Autodesk Inventor part; units mm, degrees
(part 2 of 2)
  spline S197 degree 3 poles (37.725433, 80.080162) (38.103851, 80.500583) (38.500866, 80.903886) (39.329714, 81.67384) (39.761133, 82.040107) (40.208257, 82.386568) knots 0 0 0 0 0.5 0.5 1 1 1 1
  spline S198 degree 3 poles (40.208257, 82.386568) (40.397457, 82.29423) (40.586338, 82.201241) (40.963456, 82.013963) (41.151692, 81.919675) (41.339601, 81.824739) knots 0 0 0 0 0.5 0.5 1 1 1 1
  spline S199 degree 3 poles (41.339601, 81.824739) (41.333785, 81.259123) (41.302697, 80.69405) (41.190168, 79.56837) (41.108781, 79.008326) (41.002517, 78.452752) knots 0 0 0 0 0.5 0.5 1 1 1 1
  spline S200 degree 3 poles (42.079584, 77.880352) (42.480588, 78.279289) (42.899217, 78.660108) (43.769222, 79.383234) (44.220162, 79.725179) (44.685693, 80.046483) knots 0 0 0 0 0.5 0.5 1 1 1 1
  spline S201 degree 3 poles (44.685693, 80.046483) (44.869518, 79.943863) (45.05299, 79.84061) (45.419219, 79.632841) (45.601975, 79.528327) (45.78437, 79.423183) knots 0 0 0 0 0.5 0.5 1 1 1 1
  spline S202 degree 3 poles (45.78437, 79.423183) (45.747403, 78.858747) (45.685235, 78.296245) (45.510864, 77.178473) (45.39875, 76.623762) (45.262042, 76.074886) knots 0 0 0 0 0.5 0.5 1 1 1 1
  spline S203 degree 3 poles (46.305941, 75.444022) (46.728313, 75.820263) (47.167285, 76.177443) (48.075803, 76.851543) (48.544896, 77.168128) (49.02742, 77.463299) knots 0 0 0 0 0.5 0.5 1 1 1 1
  spline S204 degree 3 poles (49.02742, 77.463299) (49.205313, 77.350708) (49.382818, 77.237505) (49.737046, 77.009877) (49.913767, 76.895453) (50.090092, 76.780422) knots 0 0 0 0 0.5 0.5 1 1 1 1
  spline S205 degree 3 poles (50.090092, 76.780422) (50.022088, 76.21888) (49.929027, 75.660656) (49.693346, 74.554187) (49.550844, 74.006495) (49.384107, 73.465983) knots 0 0 0 0 0.5 0.5 1 1 1 1
  spline S206 degree 3 poles (50.391669, 72.778571) (50.834125, 73.130973) (51.292107, 73.463428) (52.23638, 74.086457) (52.722201, 74.37672) (53.220252, 74.644861) knots 0 0 0 0 0.5 0.5 1 1 1 1
  spline S207 degree 3 poles (53.220252, 74.644861) (53.391673, 74.522642) (53.562673, 74.399832) (53.903822, 74.153036) (54.073972, 74.029051) (54.243693, 73.904481) knots 0 0 0 0 0.5 0.5 1 1 1 1
  spline S208 degree 3 poles (54.243693, 73.904481) (54.144858, 73.347538) (54.021187, 72.795288) (53.724911, 71.703483) (53.552454, 71.164472) (53.356195, 70.633966) knots 0 0 0 0 0.5 0.5 1 1 1 1
  spline S209 degree 3 poles (54.324358, 69.892093) (54.785556, 70.219586) (55.261156, 70.526308) (56.238317, 71.096373) (56.73939, 71.359432) (57.251456, 71.59973) knots 0 0 0 0 0.5 0.5 1 1 1 1
  spline S210 degree 3 poles (57.251456, 71.59973) (57.415884, 71.468253) (57.579859, 71.336209) (57.906895, 71.070995) (58.069956, 70.937825) (58.232557, 70.804095) knots 0 0 0 0 0.5 0.5 1 1 1 1
  spline S211 degree 3 poles (58.232557, 70.804095) (58.103191, 70.253442) (57.949286, 69.708844) (57.593315, 68.635017) (57.391427, 68.106325) (57.166241, 67.587436) knots 0 0 0 0 0.5 0.5 1 1 1 1
  spline S212 degree 3 poles (58.092066, 66.793356) (58.570604, 67.094946) (59.062379, 67.375002) (60.06946, 67.890371) (60.584264, 68.125428) (61.108789, 68.337152) knots 0 0 0 0 0.5 0.5 1 1 1 1
  spline S213 degree 3 poles (61.108789, 68.337152) (61.265725, 68.196817) (61.422177, 68.055941) (61.734106, 67.773114) (61.889584, 67.631164) (62.044571, 67.488679) knots 0 0 0 0 0.5 0.5 1 1 1 1
  spline S214 degree 3 poles (62.044571, 67.488679) (61.885067, 66.945988) (61.701395, 66.410695) (61.28681, 65.358109) (61.056104, 64.841342) (60.802675, 64.335645) knots 0 0 0 0 0.5 0.5 1 1 1 1
  spline S215 degree 3 poles (61.683351, 63.49177) (62.177776, 63.76654) (62.684232, 64.01908) (63.718174, 64.478189) (64.245145, 64.684529) (64.780537, 64.867037) knots 0 0 0 0 0.5 0.5 1 1 1 1
  spline S216 degree 3 poles (64.780537, 64.867037) (64.929504, 64.718269) (65.077957, 64.568989) (65.373833, 64.269408) (65.521255, 64.119108) (65.668157, 63.968302) knots 0 0 0 0 0.5 0.5 1 1 1 1
  spline S217 degree 3 poles (65.668157, 63.968302) (65.479001, 63.435222) (65.266119, 62.91086) (64.794178, 61.882711) (64.535355, 61.379437) (64.254454, 60.88847) knots 0 0 0 0 0.5 0.5 1 1 1 1
  spline S218 degree 3 poles (65.087305, 59.997361) (65.596116, 60.244477) (66.115715, 60.468734) (67.173378, 60.870188) (67.710915, 61.047185) (68.255549, 61.199923) knots 0 0 0 0 0.5 0.5 1 1 1 1
  spline S219 degree 3 poles (68.255549, 61.199923) (68.396094, 61.043175) (68.536098, 60.885943) (68.815022, 60.570518) (68.95394, 60.412325) (69.092312, 60.253656) knots 0 0 0 0 0.5 0.5 1 1 1 1
  spline S220 degree 3 poles (69.092312, 60.253656) (68.874076, 59.731805) (68.632632, 59.219967) (68.104769, 58.219377) (67.818615, 57.731125) (67.511094, 57.256377) knots 0 0 0 0 0.5 0.5 1 1 1 1
  spline S221 degree 3 poles (68.293591, 56.320742) (68.815243, 56.539453) (69.346406, 56.734746) (70.424579, 57.077327) (70.97105, 57.224444) (71.523271, 57.346946) knots 0 0 0 0 0.5 0.5 1 1 1 1
  spline S222 degree 3 poles (71.523271, 57.346946) (71.654967, 57.182694) (71.786098, 57.017989) (72.047222, 56.687677) (72.177214, 56.522072) (72.306635, 56.356021) knots 0 0 0 0 0.5 0.5 1 1 1 1
  spline S223 degree 3 poles (72.306635, 56.356021) (72.059983, 55.846985) (71.790709, 55.349224) (71.208529, 54.379233) (70.895912, 53.907486) (70.562705, 53.4504) knots 0 0 0 0 0.5 0.5 1 1 1 1
  spline S224 degree 3 poles (71.292472, 52.473079) (71.82538, 52.662721) (72.366495, 52.828457) (73.461903, 53.111124) (74.015648, 53.227913) (74.573779, 53.319809) knots 0 0 0 0 0.5 0.5 1 1 1 1
  spline S225 degree 3 poles (74.573779, 53.319809) (74.696227, 53.148551) (74.818085, 52.976872) (75.060616, 52.632678) (75.181289, 52.460163) (75.301366, 52.287234) knots 0 0 0 0 0.5 0.5 1 1 1 1
  spline S226 degree 3 poles (75.301366, 52.287234) (75.027047, 51.792559) (74.730761, 51.310388) (74.09603, 50.37394) (73.757901, 49.920131) (73.40002, 49.482095) knots 0 0 0 0 0.5 0.5 1 1 1 1
  spline S227 degree 3 poles (74.07484, 48.466057) (74.617385, 48.626055) (75.166809, 48.76173) (76.276125, 48.983624) (76.835463, 49.069731) (77.397809, 49.130742) knots 0 0 0 0 0.5 0.5 1 1 1 1
  spline S228 degree 3 poles (77.397809, 49.130742) (77.510637, 48.952998) (77.622852, 48.774867) (77.846054, 48.417835) (77.95704, 48.238934) (78.067408, 48.059654) knots 0 0 0 0 0.5 0.5 1 1 1 1
  spline S229 degree 3 poles (78.067408, 48.059654) (77.766255, 47.580841) (77.443858, 47.115724) (76.758504, 46.215664) (76.395889, 45.781171) (76.014421, 45.363514) knots 0 0 0 0 0.5 0.5 1 1 1 1
  spline S230 degree 3 poles (76.632245, 44.311845) (77.182781, 44.441712) (77.738844, 44.546915) (78.858699, 44.707362) (79.421931, 44.762526) (79.986784, 44.792465) knots 0 0 0 0 0.5 0.5 1 1 1 1
  spline S231 degree 3 poles (79.986784, 44.792465) (80.089649, 44.608777) (80.191881, 44.424734) (80.395076, 44.055948) (80.496038, 43.871206) (80.596363, 43.686117) knots 0 0 0 0 0.5 0.5 1 1 1 1
  spline S232 degree 3 poles (80.596363, 43.686117) (80.269291, 43.224621) (79.921761, 42.777971) (79.187865, 41.917032) (78.801865, 41.503174) (78.397969, 41.107166) knots 0 0 0 0 0.5 0.5 1 1 1 1
  spline S233 degree 3 poles (78.956921, 40.023059) (79.513774, 40.122402) (80.074789, 40.196812) (81.201782, 40.295325) (81.767198, 40.319378) (82.332842, 40.318156) knots 0 0 0 0 0.5 0.5 1 1 1 1
  spline S234 degree 3 poles (82.332842, 40.318156) (82.425432, 40.12908) (82.517371, 39.939685) (82.699941, 39.560265) (82.790573, 39.370242) (82.880549, 39.179907) knots 0 0 0 0 0.5 0.5 1 1 1 1
  spline S235 degree 3 poles (82.880549, 39.179907) (82.528551, 38.73713) (82.156943, 38.310302) (81.376735, 37.4911) (80.968523, 37.099134) (80.543424, 36.725977) knots 0 0 0 0 0.5 0.5 1 1 1 1
  spline S236 degree 3 poles (81.041807, 35.612725) (81.603287, 35.681241) (82.167549, 35.724633) (83.298257, 35.760913) (83.86414, 35.753782) (84.428858, 35.721402) knots 0 0 0 0 0.5 0.5 1 1 1 1
  spline S237 degree 3 poles (84.428858, 35.721402) (84.510891, 35.527512) (84.592257, 35.33334) (84.753649, 34.944439) (84.833675, 34.749711) (84.91303, 34.554709) knots 0 0 0 0 0.5 0.5 1 1 1 1
  spline S238 degree 3 poles (84.91303, 34.554709) (84.537174, 34.131995) (84.142618, 33.726287) (83.318466, 32.951308) (82.889281, 32.582425) (82.444272, 32.233253) knots 0 0 0 0 0.5 0.5 1 1 1 1
  arc A106 (84.46763, 26.481315) -> (84.09474, 27.642637) centre (0, 0) ccw
  spline S239 degree 3 poles (84.46763, 26.481315) (85.03324, 26.487647) (85.598851, 26.468703) (86.726688, 26.380376) (87.288351, 26.311036) (87.846079, 26.216729) knots 0 0 0 0 0.5 0.5 1 1 1 1
  spline S240 degree 3 poles (87.846079, 26.216729) (87.906286, 26.014991) (87.965797, 25.813047) (88.083427, 25.408752) (88.141546, 25.206402) (88.198967, 25.003854) knots 0 0 0 0 0.5 0.5 1 1 1 1
  spline S241 degree 3 poles (88.198967, 25.003854) (87.778891, 24.625053) (87.342098, 24.265211) (86.437694, 23.5856) (85.970534, 23.26617) (85.489814, 22.968071) knots 0 0 0 0 0.5 0.5 1 1 1 1
  arc A107 (85.798164, 21.787971) -> (85.489814, 22.968071) centre (0, 0) ccw
  spline S242 degree 3 poles (85.798164, 21.787971) (86.363264, 21.763135) (86.926972, 21.713062) (88.04823, 21.562739) (88.605222, 21.462564) (89.156908, 21.337675) knots 0 0 0 0 0.5 0.5 1 1 1 1
  spline S243 degree 3 poles (89.156908, 21.337675) (89.205909, 21.132927) (89.254206, 20.928011) (89.349385, 20.51785) (89.396269, 20.312606) (89.442445, 20.107203) knots 0 0 0 0 0.5 0.5 1 1 1 1
  spline S244 degree 3 poles (89.442445, 20.107203) (89.002139, 19.752118) (88.546187, 19.416884) (87.605718, 18.788126) (87.121671, 18.494916) (86.625259, 18.223752) knots 0 0 0 0 0.5 0.5 1 1 1 1
  arc A108 (86.868131, 17.028457) -> (86.625259, 18.223752) centre (0, 0) ccw
  spline S245 degree 3 poles (86.868131, 17.028457) (87.431005, 16.97253) (87.991099, 16.891479) (89.102374, 16.679616) (89.653001, 16.54891) (90.196969, 16.39382) knots 0 0 0 0 0.5 0.5 1 1 1 1
  spline S246 degree 3 poles (90.196969, 16.39382) (90.234617, 16.186684) (90.271552, 15.979418) (90.343992, 15.564637) (90.379498, 15.357122) (90.414289, 15.149487) knots 0 0 0 0 0.5 0.5 1 1 1 1
  spline S247 degree 3 poles (90.414289, 15.149487) (89.955091, 14.819196) (89.481364, 14.509589) (88.507686, 13.933594) (88.008221, 13.667494) (87.497626, 13.424088) knots 0 0 0 0 0.5 0.5 1 1 1 1
  arc A109 (87.674283, 12.217229) -> (87.497626, 13.424088) centre (0, 0) ccw
  spline S248 degree 3 poles (87.674283, 12.217229) (88.233221, 12.130379) (88.787999, 12.018597) (89.885916, 11.745838) (90.428506, 11.584998) (90.963105, 11.400177) knots 0 0 0 0 0.5 0.5 1 1 1 1
  spline S249 degree 3 poles (90.963105, 11.400177) (90.989286, 11.191281) (91.014746, 10.982296) (91.064227, 10.564154) (91.088248, 10.354998) (91.111547, 10.145762) knots 0 0 0 0 0.5 0.5 1 1 1 1
  arc A110 (88.214171, 7.368898) -> (88.104265, 8.583655) centre (0, 0) ccw
  spline S250 degree 3 poles (88.214171, 7.368898) (88.767476, 7.251389) (89.315254, 7.109215) (90.396478, 6.776388) (90.929384, 6.585902) (91.452989, 6.371912) knots 0 0 0 0 0.5 0.5 1 1 1 1
  spline S251 degree 3 poles (91.452989, 6.371912) (91.467622, 6.161892) (91.481532, 5.951821) (91.507903, 5.531588) (91.520365, 5.321427) (91.532103, 5.111224) knots 0 0 0 0 0.5 0.5 1 1 1 1
  spline S252 degree 3 poles (91.532103, 5.111224) (91.039358, 4.833454) (90.534446, 4.57784) (89.503314, 4.112454) (88.977608, 3.902914) (88.443334, 3.717155) knots 0 0 0 0 0.5 0.5 1 1 1 1
  arc A111 (88.486155, 2.498187) -> (88.443334, 3.717155) centre (0, 0) ccw
  spline S253 degree 3 poles (88.486155, 2.498187) (89.032147, 2.350376) (89.571261, 2.178242) (90.632508, 1.786359) (91.154111, 1.566805) (91.665134, 1.324296) knots 0 0 0 0 0.5 0.5 1 1 1 1
  spline S254 degree 3 poles (91.665134, 1.324296) (91.668175, 1.113788) (91.670491, 0.903271) (91.673673, 0.482223) (91.674539, 0.271694) (91.674679, 0.061164) knots 0 0 0 0 0.5 0.5 1 1 1 1
  spline S255 degree 3 poles (91.674679, 0.061164) (91.16738, -0.18904) (90.649154, -0.416451) (89.593951, -0.824328) (89.057499, -1.00459) (88.513804, -1.160635) knots 0 0 0 0 0.5 0.5 1 1 1 1
  arc A112 (88.48941, -2.380111) -> (88.513804, -1.160635) centre (0, 0) ccw
  spline S256 degree 3 poles (88.48941, -2.380111) (89.02643, -2.557774) (89.555243, -2.759345) (90.593291, -3.209095) (91.102007, -3.45705) (91.598894, -3.727342) knots 0 0 0 0 0.5 0.5 1 1 1 1
  spline S257 degree 3 poles (91.598894, -3.727342) (91.590335, -3.937697) (91.58105, -4.148023) (91.561033, -4.568607) (91.550299, -4.778863) (91.538842, -4.989081) knots 0 0 0 0 0.5 0.5 1 1 1 1
  spline S258 degree 3 poles (91.538842, -4.989081) (91.01853, -5.210959) (90.488564, -5.409478) (89.412493, -5.758606) (88.866926, -5.909042) (88.315461, -6.0349) knots 0 0 0 0 0.5 0.5 1 1 1 1
  arc A113 (88.223925, -7.25118) -> (88.315461, -6.0349) centre (0, 0) ccw
  spline S259 degree 3 poles (88.223925, -7.25118) (88.750343, -7.458157) (89.267248, -7.688553) (90.278944, -8.194804) (90.773229, -8.470406) (91.254472, -8.76766) knots 0 0 0 0 0.5 0.5 1 1 1 1
  spline S260 degree 3 poles (91.254472, -8.76766) (91.234337, -8.977224) (91.213481, -9.186719) (91.170324, -9.605561) (91.148025, -9.814908) (91.125005, -10.024175) knots 0 0 0 0 0.5 0.5 1 1 1 1
  arc A114 (87.690508, -12.100227) -> (87.848906, -10.890837) centre (0, 0) ccw
  spline S261 degree 3 poles (87.690508, -12.100227) (88.204723, -12.33589) (88.708152, -12.594411) (89.690424, -13.155625) (90.168776, -13.458037) (90.632913, -13.78135) knots 0 0 0 0 0.5 0.5 1 1 1 1
  arc A115 (86.890777, -16.912527) -> (87.115557, -15.713699) centre (0, 0) ccw
  spline S262 degree 3 poles (86.890777, -16.912527) (87.391229, -17.176158) (87.879653, -17.46202) (88.829516, -18.076493) (89.290483, -18.404798) (89.736105, -18.753188) knots 0 0 0 0 0.5 0.5 1 1 1 1
  arc A116 (85.827161, -21.673464) -> (86.117641, -20.488839) centre (0, 0) ccw
  spline S263 degree 3 poles (85.827161, -21.673464) (86.312331, -21.964264) (86.784265, -22.276597) (87.698837, -22.942463) (88.141018, -23.295663) (88.566771, -23.668073) knots 0 0 0 0 0.5 0.5 1 1 1 1
  arc A117 (84.502891, -26.368579) -> (84.858189, -25.201755) centre (0, 0) ccw
  spline S264 degree 3 poles (84.502891, -26.368579) (84.971305, -26.685664) (85.425317, -27.023522) (86.301819, -27.738758) (86.723871, -28.11578) (87.128462, -28.511078) knots 0 0 0 0 0.5 0.5 1 1 1 1
  arc A118 (82.921989, -30.983614) -> (83.341025, -29.838134) centre (0, 0) ccw
  spline S265 degree 3 poles (82.921989, -30.983614) (83.372224, -31.326022) (83.806935, -31.688376) (84.642705, -32.450811) (85.043347, -32.850511) (85.425548, -33.267496) knots 0 0 0 0 0.5 0.5 1 1 1 1
  arc A119 (81.089256, -35.504553) -> (81.570757, -34.383896) centre (0, 0) ccw
  spline S266 degree 3 poles (81.089256, -35.504553) (81.519944, -35.871243) (81.934034, -36.256994) (82.726534, -37.064312) (83.104549, -37.485475) (83.463199, -37.922882) knots 0 0 0 0 0.5 0.5 1 1 1 1
  arc A120 (79.010257, -39.917665) -> (79.552761, -38.825235) centre (0, 0) ccw
  spline S267 degree 3 poles (79.010257, -39.917665) (79.420091, -40.307524) (79.812301, -40.715501) (80.559125, -41.56525) (80.913365, -42.006598) (81.247375, -42.463098) knots 0 0 0 0 0.5 0.5 1 1 1 1
  arc A121 (76.691306, -44.209549) -> (77.293166, -43.148663) centre (0, 0) ccw
  spline S268 degree 3 poles (76.691306, -44.209549) (77.079042, -44.621393) (77.448182, -45.050356) (78.147061, -45.939956) (78.47645, -46.400147) (78.784805, -46.874354) knots 0 0 0 0 0.5 0.5 1 1 1 1
  arc A122 (74.139446, -48.36717) -> (74.798835, -47.341049) centre (0, 0) ccw
  spline S269 degree 3 poles (74.139446, -48.36717) (74.503906, -48.799748) (74.848855, -49.248395) (75.497666, -50.175143) (75.801205, -50.652781) (76.082968, -51.143255) knots 0 0 0 0 0.5 0.5 1 1 1 1
  arc A123 (71.362428, -52.377901) -> (72.077341, -51.389663) centre (0, 0) ccw
  spline S270 degree 3 poles (71.362428, -52.377901) (71.702504, -52.829899) (72.022214, -53.296868) (72.618988, -54.25795) (72.895754, -54.751584) (73.15007, -55.256835) knots 0 0 0 0 0.5 0.5 1 1 1 1
  arc A124 (68.368684, -56.229562) -> (69.136952, -55.282208) centre (0, 0) ccw
  spline S271 degree 3 poles (68.368684, -56.229562) (68.683345, -56.699608) (68.976845, -57.18348) (69.519768, -58.175978) (69.768921, -58.684109) (69.995018, -59.202602) knots 0 0 0 0 0.5 0.5 1 1 1 1
  arc A125 (65.167307, -59.910456) -> (65.986595, -59.006863) centre (0, 0) ccw
  spline S272 degree 3 poles (65.167307, -59.910456) (65.455596, -60.397123) (65.721995, -60.896428) (66.209419, -61.917327) (66.430201, -62.438412) (66.627393, -62.968572) knots 0 0 0 0 0.5 0.5 1 1 1 1
  arc A126 (61.768018, -63.409404) -> (62.63584, -62.552316) centre (0, 0) ccw
  spline S273 degree 3 poles (61.768018, -63.409404) (62.02906, -63.911213) (62.267549, -64.424435) (62.697995, -65.470635) (62.889736, -66.003091) (63.057422, -66.543309) knots 0 0 0 0 0.5 0.5 1 1 1 1
  arc A127 (58.181142, -66.71578) -> (59.094861, -65.907799) centre (0, 0) ccw
  spline S274 degree 3 poles (58.181142, -66.71578) (58.414144, -67.231207) (58.623999, -67.756787) (58.996158, -68.825111) (59.158277, -69.367321) (59.295949, -69.915957) knots 0 0 0 0 0.5 0.5 1 1 1 1
  arc A128 (54.417572, -69.819542) -> (55.374414, -69.063123) centre (0, 0) ccw
  spline S275 degree 3 poles (54.417572, -69.819542) (54.621827, -70.347021) (54.80241, -70.883364) (55.115152, -71.970568) (55.247155, -72.520885) (55.354396, -73.076271) knots 0 0 0 0 0.5 0.5 1 1 1 1
  arc A129 (50.488738, -72.711264) -> (51.485796, -72.008704) centre (0, 0) ccw
  spline S276 degree 3 poles (50.488738, -72.711264) (50.663625, -73.249195) (50.814388, -73.794671) (51.066763, -74.897452) (51.16825, -75.454205) (51.244733, -76.014656) knots 0 0 0 0 0.5 0.5 1 1 1 1
  arc A130 (46.406571, -75.382165) -> (47.440817, -74.735597) centre (0, 0) ccw
  spline S277 degree 3 poles (46.406571, -75.382165) (46.551559, -75.928913) (46.672044, -76.481866) (46.863286, -77.596875) (46.933949, -78.158374) (46.979441, -78.722186) knots 0 0 0 0 0.5 0.5 1 1 1 1
  arc A131 (42.183469, -77.824132) -> (43.251763, -77.235521) centre (0, 0) ccw
  spline S278 degree 3 poles (42.183469, -77.824132) (42.298117, -78.378037) (42.387958, -78.936788) (42.517487, -80.060639) (42.557111, -80.625177) (42.571475, -81.19064) knots 0 0 0 0 0.5 0.5 1 1 1 1
  arc A132 (37.832257, -80.029751) -> (38.931354, -79.500883) centre (0, 0) ccw
  spline S279 degree 3 poles (37.832257, -80.029751) (37.916218, -80.58913) (37.975142, -81.151981) (38.042564, -82.281261) (38.051028, -82.847125) (38.03422, -83.412521) knots 0 0 0 0 0.5 0.5 1 1 1 1
  arc A133 (33.366149, -81.992321) -> (34.492711, -81.524803) centre (0, 0) ccw
  spline S280 degree 3 poles (33.366149, -81.992321) (33.419168, -82.555476) (33.446996, -83.120719) (33.452106, -84.251998) (33.429386, -84.817469) (33.381457, -85.38108) knots 0 0 0 0 0.5 0.5 1 1 1 1
  arc A134 (28.79871, -83.705883) -> (29.949316, -83.301135) centre (0, 0) ccw
  spline S281 degree 3 poles (28.79871, -83.705883) (28.820625, -84.271104) (28.817273, -84.837022) (28.760056, -85.966864) (28.706219, -86.530225) (28.627315, -87.09034) knots 0 0 0 0 0.5 0.5 1 1 1 1
  arc A135 (24.14381, -85.165234) -> (25.314966, -84.824484) centre (0, 0) ccw
  spline S282 degree 3 poles (24.14381, -85.165234) (24.134555, -85.730803) (24.100033, -86.295677) (23.980662, -87.420652) (23.895873, -87.980192) (23.786233, -88.53511) knots 0 0 0 0 0.5 0.5 1 1 1 1
  arc A136 (19.415586, -86.36594) -> (20.603734, -86.090224) centre (0, 0) ccw
  spline S283 degree 3 poles (19.415586, -86.36594) (19.375189, -86.930141) (19.309602, -87.492255) (19.12844, -88.608946) (19.012956, -89.162966) (18.872913, -89.711001) knots 0 0 0 0 0.5 0.5 1 1 1 1
  arc A137 (14.628398, -87.304356) -> (15.82993, -87.094511) centre (0, 0) ccw
  spline S284 degree 3 poles (14.628398, -87.304356) (14.556982, -87.865475) (14.460528, -88.423123) (14.218126, -89.528138) (14.072297, -90.074954) (13.902277, -90.614443) knots 0 0 0 0 0.5 0.5 1 1 1 1
  arc A138 (9.796783, -87.977632) -> (11.008051, -87.834295) centre (0, 0) ccw
  spline S285 degree 3 poles (9.796783, -87.977632) (9.694565, -88.533964) (9.567539, -89.085452) (9.264631, -90.175436) (9.088901, -90.713388) (8.88942, -91.242691) knots 0 0 0 0 0.5 0.5 1 1 1 1
  arc A139 (4.935416, -88.383722) -> (6.152741, -88.307329) centre (0, 0) ccw
  spline S286 degree 3 poles (4.935416, -88.383722) (4.802706, -88.933579) (4.645492, -89.477231) (4.283, -90.548874) (4.077902, -91.076329) (3.849566, -91.593839) knots 0 0 0 0 0.5 0.5 1 1 1 1
  spline S287 degree 3 poles (86.687632, 29.82457) (86.289061, 29.423203) (85.872755, 29.039845) (85.007162, 28.311444) (84.558308, 27.966765) (84.09474, 27.642637) knots 0 0 0 0 0.5 0.5 1 1 1 1
  spline S288 degree 3 poles (91.111547, 10.145762) (90.634852, 9.841269) (90.144788, 9.558228) (89.140859, 9.036746) (88.627494, 8.798565) (88.104265, 8.583655) knots 0 0 0 0 0.5 0.5 1 1 1 1
  spline S289 degree 3 poles (91.125005, -10.024175) (90.59326, -10.217054) (90.053162, -10.386076) (88.959493, -10.675396) (88.406468, -10.79555) (87.848906, -10.890837) knots 0 0 0 0 0.5 0.5 1 1 1 1
  spline S290 degree 3 poles (90.632913, -13.78135) (90.601264, -13.989488) (90.568899, -14.197516) (90.502735, -14.613345) (90.468937, -14.821144) (90.434423, -15.028826) knots 0 0 0 0 0.5 0.5 1 1 1 1
  spline S291 degree 3 poles (89.736105, -18.753188) (89.693038, -18.959266) (89.649262, -19.165195) (89.560292, -19.576747) (89.515098, -19.78237) (89.469196, -19.987835) knots 0 0 0 0 0.5 0.5 1 1 1 1
  spline S292 degree 3 poles (88.566771, -23.668073) (88.512417, -23.871465) (88.457363, -24.07467) (88.345857, -24.480696) (88.289404, -24.683517) (88.232253, -24.886141) knots 0 0 0 0 0.5 0.5 1 1 1 1
  spline S293 degree 3 poles (87.128462, -28.511078) (87.062987, -28.711167) (86.996823, -28.911031) (86.863118, -29.310298) (86.795578, -29.509701) (86.727352, -29.708869) knots 0 0 0 0 0.5 0.5 1 1 1 1
  spline S294 degree 3 poles (85.425548, -33.267496) (85.349149, -33.463675) (85.272075, -33.65959) (85.116579, -34.050886) (85.038157, -34.246265) (84.959063, -34.441372) knots 0 0 0 0 0.5 0.5 1 1 1 1
  spline S295 degree 3 poles (83.463199, -37.922882) (83.376109, -38.114554) (83.28836, -38.305926) (83.111544, -38.688062) (83.022478, -38.878824) (82.932756, -39.069278) knots 0 0 0 0 0.5 0.5 1 1 1 1
  spline S296 degree 3 poles (81.247375, -42.463098) (81.149859, -42.649681) (81.0517, -42.835928) (80.854102, -43.207743) (80.754663, -43.39331) (80.654585, -43.578532) knots 0 0 0 0 0.5 0.5 1 1 1 1
  spline S297 degree 3 poles (78.784805, -46.874354) (78.677158, -47.055282) (78.568889, -47.235839) (78.351108, -47.596204) (78.241598, -47.776011) (78.131469, -47.955439) knots 0 0 0 0 0.5 0.5 1 1 1 1
  spline S298 degree 3 poles (76.082968, -51.143255) (75.965518, -51.317978) (75.847467, -51.492297) (75.610165, -51.840117) (75.490916, -52.013618) (75.37107, -52.186707) knots 0 0 0 0 0.5 0.5 1 1 1 1
  spline S299 degree 3 poles (73.15007, -55.256835) (73.023173, -55.424823) (72.895698, -55.592374) (72.639597, -55.926594) (72.51097, -56.093262) (72.381771, -56.259486) knots 0 0 0 0 0.5 0.5 1 1 1 1
  spline S300 degree 3 poles (69.995018, -59.202602) (69.85906, -59.363344) (69.722548, -59.523618) (69.448424, -59.843223) (69.310811, -60.002552) (69.172651, -60.161407) knots 0 0 0 0 0.5 0.5 1 1 1 1
  spline S301 degree 3 poles (66.627393, -62.968572) (66.482786, -63.121581) (66.337653, -63.274092) (66.046338, -63.57811) (65.900158, -63.729617) (65.753457, -63.880619) knots 0 0 0 0 0.5 0.5 1 1 1 1
  spline S302 degree 3 poles (63.057422, -66.543309) (62.904607, -66.68812) (62.751292, -66.832404) (62.443672, -67.119912) (62.289368, -67.263137) (62.134571, -67.405828) knots 0 0 0 0 0.5 0.5 1 1 1 1
  spline S303 degree 3 poles (59.295949, -69.915957) (59.135388, -70.052129) (58.974358, -70.187748) (58.651367, -70.457874) (58.489407, -70.59238) (58.326985, -70.726328) knots 0 0 0 0 0.5 0.5 1 1 1 1
  spline S304 degree 3 poles (55.354396, -73.076271) (55.186577, -73.203392) (55.018321, -73.329934) (54.680939, -73.581857) (54.511815, -73.707237) (54.342261, -73.832034) knots 0 0 0 0 0.5 0.5 1 1 1 1
  spline S305 degree 3 poles (51.244733, -76.014656) (51.070166, -76.132339) (50.895194, -76.24942) (50.544448, -76.482375) (50.368673, -76.598248) (50.192502, -76.713514) knots 0 0 0 0 0.5 0.5 1 1 1 1
  spline S306 degree 3 poles (46.979441, -78.722186) (46.798657, -78.830074) (46.617501, -78.937339) (46.254454, -79.150618) (46.072564, -79.256632) (45.89031, -79.362019) knots 0 0 0 0 0.5 0.5 1 1 1 1
  spline S307 degree 3 poles (42.571475, -81.19064) (42.385021, -81.288405) (42.198232, -81.385527) (41.823987, -81.578484) (41.636533, -81.674317) (41.44875, -81.769503) knots 0 0 0 0 0.5 0.5 1 1 1 1
  spline S308 degree 3 poles (38.03422, -83.412521) (37.842664, -83.499866) (37.650808, -83.586551) (37.266502, -83.758598) (37.074053, -83.843959) (36.881312, -83.928656) knots 0 0 0 0 0.5 0.5 1 1 1 1
  spline S309 degree 3 poles (33.381457, -85.38108) (33.18538, -85.45774) (32.98904, -85.533725) (32.59584, -85.68434) (32.398981, -85.75897) (32.201867, -85.832921) knots 0 0 0 0 0.5 0.5 1 1 1 1
  spline S310 degree 3 poles (28.627315, -87.09034) (28.427313, -87.156083) (28.227085, -87.221136) (27.826185, -87.349861) (27.625514, -87.413533) (27.424625, -87.476514) knots 0 0 0 0 0.5 0.5 1 1 1 1
  spline S311 degree 3 poles (23.786233, -88.53511) (23.582913, -88.589734) (23.379406, -88.643659) (22.972023, -88.750104) (22.768149, -88.802625) (22.564096, -88.854443) knots 0 0 0 0 0.5 0.5 1 1 1 1
  spline S312 degree 3 poles (18.872913, -89.711001) (18.666893, -89.754342) (18.460724, -89.796974) (18.048096, -89.880816) (17.841639, -89.922026) (17.635041, -89.962525) knots 0 0 0 0 0.5 0.5 1 1 1 1
  spline S313 degree 3 poles (13.902277, -90.614443) (13.694182, -90.646369) (13.485978, -90.677579) (13.069358, -90.738563) (12.860943, -90.768337) (12.652428, -90.797393) knots 0 0 0 0 0.5 0.5 1 1 1 1
  spline S314 degree 3 poles (8.88942, -91.242691) (8.679882, -91.263106) (8.470275, -91.282799) (8.050928, -91.320739) (7.84119, -91.338987) (7.631391, -91.356513) knots 0 0 0 0 0.5 0.5 1 1 1 1
  spline S315 degree 3 poles (3.849566, -91.593839) (3.639222, -91.60268) (3.428848, -91.610796) (3.008048, -91.625578) (2.797623, -91.632244) (2.587177, -91.638186) knots 0 0 0 0 0.5 0.5 1 1 1 1
  spline S316 degree 3 poles (2.587177, -91.638186) (2.323089, -91.137973) (2.081485, -90.62621) (1.644687, -89.582646) (1.449713, -89.051366) (1.278745, -88.512177) knots 0 0 0 0 0.5 0.5 1 1 1 1
  spline S317 degree 3 poles (90.434423, -15.028826) (89.892861, -15.192119) (89.344272, -15.331132) (88.236326, -15.559765) (87.677521, -15.649271) (87.115557, -15.713699) knots 0 0 0 0 0.5 0.5 1 1 1 1
  spline S318 degree 3 poles (89.469196, -19.987835) (88.91946, -20.121046) (88.364047, -20.229628) (87.245188, -20.396879) (86.682301, -20.455466) (86.117641, -20.488839) knots 0 0 0 0 0.5 0.5 1 1 1 1
  spline S319 degree 3 poles (88.232253, -24.886141) (87.676014, -24.988867) (87.115462, -25.066687) (85.989089, -25.172049) (85.42383, -25.199539) (84.858189, -25.201755) knots 0 0 0 0 0.5 0.5 1 1 1 1
  spline S320 degree 3 poles (86.727352, -29.708869) (86.166299, -29.780797) (85.602311, -29.827619) (84.471844, -29.870772) (83.905929, -29.867081) (83.341025, -29.838134) knots 0 0 0 0 0.5 0.5 1 1 1 1
  spline S321 degree 3 poles (84.959063, -34.441372) (84.394899, -34.482284) (83.829189, -34.497966) (82.698061, -34.478778) (82.133208, -34.443918) (81.570757, -34.383896) knots 0 0 0 0 0.5 0.5 1 1 1 1
  spline S322 degree 3 poles (82.932756, -39.069278) (82.367195, -39.079049) (81.80148, -39.063544) (80.673127, -38.982074) (80.111052, -38.91615) (79.552761, -38.825235) knots 0 0 0 0 0.5 0.5 1 1 1 1
  spline S323 degree 3 poles (80.654585, -43.578532) (80.089345, -43.557132) (79.525343, -43.510487) (78.403191, -43.366982) (77.845601, -43.270195) (77.293166, -43.148663) knots 0 0 0 0 0.5 0.5 1 1 1 1
  spline S324 degree 3 poles (78.131469, -47.955439) (77.568265, -47.902934) (77.00769, -47.82529) (75.895147, -47.620186) (75.343736, -47.49283) (74.798835, -47.341049) knots 0 0 0 0 0.5 0.5 1 1 1 1
  spline S325 degree 3 poles (75.37107, -52.186707) (74.811614, -52.103256) (74.256167, -51.994849) (73.156612, -51.728769) (72.613054, -51.57123) (72.077341, -51.389663) knots 0 0 0 0 0.5 0.5 1 1 1 1
  spline S326 degree 3 poles (72.381771, -56.259486) (71.827762, -56.145343) (71.27913, -56.006502) (70.195903, -55.680254) (69.661849, -55.493011) (69.136952, -55.282208) knots 0 0 0 0 0.5 0.5 1 1 1 1
  spline S327 degree 3 poles (69.172651, -60.161407) (68.625772, -60.016917) (68.085621, -59.848064) (67.022011, -59.46264) (66.499083, -59.246261) (65.986595, -59.006863) knots 0 0 0 0 0.5 0.5 1 1 1 1
  spline S328 degree 3 poles (65.753457, -63.880619) (65.215367, -63.706223) (64.685338, -63.50787) (63.644576, -63.064439) (63.134361, -62.819582) (62.63584, -62.552316) knots 0 0 0 0 0.5 0.5 1 1 1 1
  spline S329 degree 3 poles (62.134571, -67.405828) (61.606905, -67.202054) (61.088608, -66.974805) (60.073854, -66.474714) (59.577902, -66.202122) (59.094861, -65.907799) knots 0 0 0 0 0.5 0.5 1 1 1 1
  spline S330 degree 3 poles (58.326985, -70.726328) (57.811346, -70.493796) (57.306354, -70.23834) (56.320689, -69.683107) (55.840508, -69.383608) (55.374414, -69.063123) knots 0 0 0 0 0.5 0.5 1 1 1 1
  spline S331 degree 3 poles (54.342261, -73.832034) (53.840215, -73.57145) (53.350063, -73.288562) (52.396481, -72.679875) (51.933527, -72.354379) (51.485796, -72.008704) knots 0 0 0 0 0.5 0.5 1 1 1 1
  spline S332 degree 3 poles (50.192502, -76.713514) (49.705573, -76.425669) (49.231749, -76.11621) (48.313146, -75.455917) (47.868826, -75.105412) (47.440817, -74.735597) knots 0 0 0 0 0.5 0.5 1 1 1 1
  spline S333 degree 3 poles (45.89031, -79.362019) (45.419977, -79.047787) (44.96392, -78.712696) (44.083086, -78.002801) (43.658749, -77.628352) (43.251763, -77.235521) knots 0 0 0 0 0.5 0.5 1 1 1 1
  spline S334 degree 3 poles (41.44875, -81.769503) (40.996442, -81.429839) (40.559537, -81.070134) (39.719147, -80.312794) (39.316082, -79.915537) (38.931354, -79.500883) knots 0 0 0 0 0.5 0.5 1 1 1 1
  spline S335 degree 3 poles (36.881312, -83.928656) (36.448402, -83.564591) (36.031975, -83.181364) (35.234582, -82.378879) (34.854014, -81.960022) (34.492711, -81.524803) knots 0 0 0 0 0.5 0.5 1 1 1 1
  spline S336 degree 3 poles (32.201867, -85.832921) (31.789669, -85.445561) (31.394986, -85.039975) (30.643011, -84.194782) (30.286094, -83.755596) (29.949316, -83.301135) knots 0 0 0 0 0.5 0.5 1 1 1 1
  spline S337 degree 3 poles (27.424625, -87.476514) (27.034393, -87.067035) (26.662652, -86.640323) (25.958378, -85.754989) (25.626197, -85.296808) (25.314966, -84.824484) knots 0 0 0 0 0.5 0.5 1 1 1 1
  spline S338 degree 3 poles (22.564096, -88.854443) (22.197013, -88.424089) (21.849344, -87.977547) (21.194911, -87.05476) (20.888474, -86.578976) (20.603734, -86.090224) knots 0 0 0 0 0.5 0.5 1 1 1 1
  spline S339 degree 3 poles (17.635041, -89.962525) (17.292223, -89.512602) (16.96968, -89.047586) (16.367075, -88.090149) (16.087313, -87.598206) (15.82993, -87.094511) knots 0 0 0 0 0.5 0.5 1 1 1 1
  spline S340 degree 3 poles (12.652428, -90.797393) (12.334916, -90.329269) (12.03848, -89.84719) (11.489533, -88.858011) (11.237296, -88.351404) (11.008051, -87.834295) knots 0 0 0 0 0.5 0.5 1 1 1 1
  spline S341 degree 3 poles (7.631391, -91.356513) (7.340148, -90.871608) (7.070719, -90.373932) (6.577097, -89.356014) (6.353151, -88.836281) (6.152741, -88.307329) knots 0 0 0 0 0.5 0.5 1 1 1 1
  point P0 (86.09924, -40.148735)
  point P1 (86.09924, 40.148735)
  dimension "d0" = 15
  dimension "d1" = 25
  constraints: 6 end point, 1 centre point, 1 coincident, 1 horizontal, 1 point on circle, 1 symmetric about line
  measures "d0" radial gap between concentric circles of A86 A93
  measures "d1" angle of L9 L8
extrude "Extrusion1" add sketch "Sketch1" along normal blind 5 contours A86 L9 A93 L8 | A86 L10 A93 L9 | A98 L15 A99 L16 | L21 A104 L22 A105
ref_plane "Work Plane1" through (0, 0, 0) normal (0, -1, 0) x (1, 0, 0)
sketch "Sketch2" plane through (0, 0, 0) normal (0, -1, 0) x (1, 0, 0)
  line L0 (95, 5) -> (95, 0)
  line L1 (110, 0) -> (110, 5)
  line L2 (99.693857, 5) -> (99.693857, 5)
  line L3 (99.693857, 5) -> (86.09924, 5)
  line L4 (86.09924, 5) -> (86.09924, 5)
  line L5 (86.09924, 5) -> (99.693857, 5)
  line L6 (86.09924, 5) -> (95, 5)
  line L7 (110, 0) -> (95, 0)
  line L8 (95, 0) -> (95, 5)
  line L9 (95, 5) -> (110, 5)
  line L10 (110, 5) -> (110, 0)
  line L11 (98.236117, 6.076619) -> (101.70908, 25.772774)
  line L12 (101.70908, 25.772774) -> (107.814888, 24.696155)
  line L13 (107.814888, 24.696155) -> (104.341925, 5)
  line L14 (104.341925, 5) -> (98.236117, 6.076619)
  line L15 (106.775404, 1.524632) -> (111.290256, 27.129634)
  line L16 (111.290256, 27.129634) -> (99.275602, 29.248142)
  line L17 (99.275602, 29.248142) -> (94.760749, 3.64314)
  line L18 (94.760749, 3.64314) -> (106.775404, 1.524632)
  line L19 (107.814888, 24.696155) -> (110.769312, 24.175211)
  line L20 (101.70908, 25.772774) -> (98.754657, 26.293718)
  point P0 (0, 0)
  point P1 (107.388205, 5)
  dimension "d5" = 6.2
  dimension "d6" = 80
  dimension "d7" = 3
  dimension "d8" = 20
  constraints: 28 end point, 6 parallel, 6 point on line, 3 perpendicular, 1 horizontal, 3 other
  measures "d5" distance of L11.end L12.end
  measures "d6" angle of L9 L13
  measures "d7" distance between parallel lines of L13 L15
  measures "d8" distance of L12.end L13.end
extrude "Extrusion2" add sketch "Sketch2" along normal mid plane 50 contours L17 L20 L11 L14 L9 L3 | L13 L19 L15 L9
sketch "Sketch3" plane through (0, 25, 0) normal (0, 1, 0) x (1, 0, 0)
  line L0 (104.341925, -5) -> (107.814888, -24.696155)
  line L1 (107.814888, -24.696155) -> (110.769312, -24.175211)
  line L2 (110.769312, -24.175211) -> (107.388205, -5)
  line L3 (104.341925, -5) -> (107.121426, -5)
  line L4 (98.754657, -26.293718) -> (101.70908, -25.772774)
  line L5 (101.70908, -25.772774) -> (98.236117, -6.076619)
  line L6 (98.236117, -6.076619) -> (104.341925, -5)
  line L7 (95, -5) -> (104.341925, -5)
  line L8 (95, -5) -> (98.754657, -26.293718)
  line L9 (110.769312, -24.175211) -> (107.388205, -5)
  line L10 (95, -5) -> (98.754657, -26.293718)
  line L11 (110.769312, -24.175211) -> (98.754657, -26.293718)
  line L12 (98.754657, -26.293718) -> (95, -5)
  line L13 (95, -5) -> (107.014655, -2.881492)
  line L14 (107.014655, -2.881492) -> (110.769312, -24.175211)
  line L15 (107.388205, -5) -> (107.121426, -5)
  point P0 (0, 0)
  point P1 (106.169693, -5)
  point P2 (107.814888, -24.696155)
  constraints: 8 end point, 2 parallel, 2 perpendicular, 1 other
extrude "Extrusion3" add sketch "Sketch3" against normal blind 3 contours L0 L11 L5 L6
mirror "Mirror1" about plane through (0, 0, 0) normal (0, -1, 0) of "Extrusion3"
chamfer "Chamfer1" distance 5 angle 45 2 edges at (92.8965, 43.3184, 5) (92.8965, -43.3184, 5)
chamfer "Chamfer2" distance 2.25 angle 45 3 edges at (101.0607, 25, 5) (101.0607, -25, 5) (107.3882, 0, 5)
sketch "Sketch4" plane through (110.769312, -25, 24.175211) normal (0.9848078, 0, -0.1736482) x (-0.1736482, 0, -0.9848078)
  circle A0 centre (10, 39) radius 1.5 projected
  circle A1 centre (10, 11) radius 1.5 projected
  point P0 (43.042824, 25)
extrude "Extrusion4" cut sketch "Sketch4" against normal through all
sketch "Sketch5" plane through (0, 0, 0) normal (0, 0, -1) x (-1, 0, 0)
  arc A0 (-105.234033, -12.72) -> (-97.582335, -41.396714) centre (0, 0) ccw
  arc A1 (-99.277389, -12) -> (-92.058806, -39.053504) centre (0, 0) ccw
  line L0 (-97.582335, -41.396714) -> (-92.058806, -39.053504)
  line L1 (-99.277389, -12) -> (-105.234033, -12.72)
  arc A2 (-92.058806, 39.053504) -> (-99.277389, 12) centre (0, 0) ccw
  arc A3 (-97.582335, 41.396714) -> (-105.234033, 12.72) centre (0, 0) ccw
  line L2 (-92.058806, 39.053504) -> (-97.582335, 41.396714)
  line L3 (-105.234033, 12.72) -> (-99.277389, 12)
  arc A4 (-97.47615, 41.134416) -> (-105.01129, 12.894532) centre (0, 0) ccw
  line L4 (-97.47615, 41.134416) -> (-92.320847, 38.947415)
  arc A5 (-92.320847, 38.947415) -> (-99.451746, 12.222531) centre (0, 0) ccw
  line L5 (-99.451746, 12.222531) -> (-105.01129, 12.894532)
  arc A6 (-105.01129, -12.894532) -> (-97.47615, -41.134416) centre (0, 0) ccw
  line L6 (-105.01129, -12.894532) -> (-99.451746, -12.222531)
  arc A7 (-99.451746, -12.222531) -> (-92.320847, -38.947415) centre (0, 0) ccw
  line L7 (-92.320847, -38.947415) -> (-97.47615, -41.134416)
  point P0 (0, 0)
  dimension "d21" = 0.2
  dimension "d22" = 0.2
  constraints: 8 end point, 8 point on circle, 4 centre point, 6 other
  measures "d21" radial gap between concentric circles of A3 A4
  measures "d22" radial gap between concentric circles of A0 A6
sketch "Sketch5 outline for Extrusion5" plane through (0, 0, 0) normal (0, 0, -1) x (-1, 0, 0)
  line L0 (-92.320847, 38.947415) -> (-97.47615, 41.134416)
  arc A0 (-99.451746, 12.222531) -> (-92.320847, 38.947415) centre (0, 0) cw
  line L1 (-105.01129, 12.894532) -> (-99.451746, 12.222531)
  arc A1 (-97.47615, 41.134416) -> (-105.01129, 12.894532) centre (0, 0) ccw
  line L2 (-99.451746, -12.222531) -> (-105.01129, -12.894532)
  arc A2 (-92.320847, -38.947415) -> (-99.451746, -12.222531) centre (0, 0) cw
  line L3 (-97.47615, -41.134416) -> (-92.320847, -38.947415)
  arc A3 (-105.01129, -12.894532) -> (-97.47615, -41.134416) centre (0, 0) ccw
extrude "Extrusion5" add sketch "Sketch5 outline for Extrusion5" along normal blind 4.5
body "Solid1"
